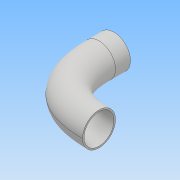
# Autodesk Inventor part: Pipe
Saved by Autodesk Inventor 2018.1 (Build 221171000, 171)
## iProperties
Created: 2019-02-11
Part Number: Pipe
Material: Generic
Document SubType Name: Modeling
Designer: James
Density: 1 g/cm^3
Appearance: Default
Author: James
Autodesk Inventor part; units mm, degrees
ref_plane "YZ Plane" through (0, 0, 0) normal (1, 0, 0) x (0, 1, 0)
ref_plane "XZ Plane" through (0, 0, 0) normal (0, 1, 0) x (-1, 0, 0)
ref_plane "XY Plane" through (0, 0, 0) normal (0, 0, 1) x (1, 0, 0)
sketch "Sketch1" plane through (0, 0, 0) normal (0, 1, 0) x (-1, 0, 0)
  circle A0 centre (0, 0) radius 20
  circle A1 centre (0, 0) radius 22
  dimension "d0" = 40
  dimension "d1" = 2
  constraints: 2 centre point, 2 coincident
  measures "d0" diameter of A0
  measures "d1" radial gap between concentric circles of A0 A1
sketch3d "3D Sketch4"
  line L0 (0, 0, 0) -> (0, -20, 0)
  spline S0 degree 2 poles (0, -20, 0) (0, -100, 0) (80, -100, 0) knots 1 1 1 2 2 2
  dimension "d4" = 20
  dimension "d5" = 80
  dimension "d6" = 80
sweep "Sweep1" add profiles "Sketch1" path "3D Sketch4"
body "Solid1"
